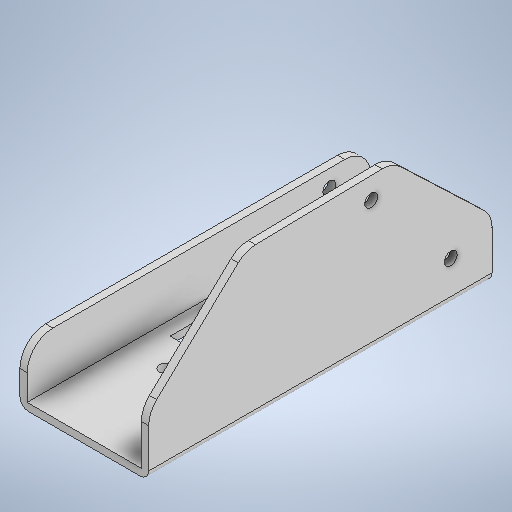
# Autodesk Inventor part: gripper servo mount
Saved by Autodesk Inventor 2025.2 (Build 292293000, 293)
## iProperties
Created: 2025-05-22
Part Number: gripper servo mount
Material: Generic
Document SubType Name: Modeling
Designer: Verchasv
Density: 1 g/cm^3
Appearance: Default
Author: Verchasv
Autodesk Inventor part; units mm, degrees
ref_plane "YZ Plane" through (0, 0, 0) normal (1, 0, 0) x (0, 1, 0)
ref_plane "XZ Plane" through (0, 0, 0) normal (0, 1, 0) x (-1, 0, 0)
ref_plane "XY Plane" through (0, 0, 0) normal (0, 0, 1) x (1, 0, 0)
sketch "Sketch1" plane through (0, 0, 0) normal (0, 1, 0) x (-1, 0, 0)
  line L0 (0, 0) -> (20, 0)
  line L1 (20, 0) -> (20, -40)
  line L2 (20, -40) -> (0, -40)
  line L3 (0, -40) -> (0, 0)
  line L4 (25, 30) -> (-5, 30)
  line L5 (-5, 30) -> (-5, -50)
  line L6 (-5, -50) -> (25, -50)
  line L7 (25, -50) -> (25, 30)
  dimension "d0" = 20
  dimension "d1" = 40
  dimension "d2" = 30
  dimension "d3" = 30
  dimension "d4" = 10
  dimension "d5" = 5
  constraints: 16 end point, 4 parallel, 2 horizontal, 2 perpendicular
  measures "d0" distance of L1.end L2.end
  measures "d1" distance of L0.end L1.end
  measures "d2" distance of L4.start L4.end
  measures "d3" distance between parallel lines of L0 L4
  measures "d4" distance between parallel lines of L2 L6
  measures "d5" distance between parallel lines of L5 L3
extrude "Extrusion1" add sketch "Sketch1" along normal blind 1.7
sketch "Sketch2" plane through (5, 0, 30) normal (1, 0, 0) x (0, 0, -1)
  line L0 (0, 0) -> (0, 1.7) projected
  line L1 (0, 1.7) -> (0, 13.7)
  line L2 (0, 13.7) -> (22.5503, 35.1708)
  line L3 (22.5503, 35.1708) -> (56.8462, 35.7913)
  line L4 (56.8462, 35.7913) -> (80, 13.7)
  line L5 (80, 0) -> (80, 1.7) projected
  line L6 (80, 13.7) -> (80, 1.7)
  line L7 (0, 1.7) -> (80, 1.7) projected
  circle A0 centre (70.3665, 9.7) radius 1.5
  circle A1 centre (70.3665, 9.7) radius 28
  line L8 (24.8863, 30.7) -> (59.3173, 30.7)
  circle A2 centre (51.8462, 30.7) radius 1.5
  point P0 (30, 0)
  dimension "d11" = 56
  dimension "d8" = 0
  dimension "d9" = 3
  dimension "d10" = 8
  dimension "d12" = 29
  dimension "d13" = 3
  dimension "d14" = 5
  dimension "d15" = 5
  dimension "d16" = 12
  dimension "d19" = 12
  constraints: 12 end point, 2 centre point, 1 coincident, 1 horizontal, 1 point on line, 1 vertical, 3 other
  measures "d8" horizontal distance of L5.end L4.end
  measures "d9" diameter of A0
  measures "d10" distance from line of L7 A0.centre
  measures "d12" distance between parallel lines of L7 L8
  measures "d13" diameter of A2
  measures "d14" horizontal distance of L3.end A2.centre
  measures "d15" distance from line of L3 A2.centre
  measures "d16" distance of L4.end L5.end
  measures "d19" distance of L0.end L1.end
extrude "Extrusion2" add sketch "Sketch2" against normal blind 1.7 contours L1 L2 L3 L4 A1 A2 L7 | A1 A2 L4 L6 L7
sketch "Sketch3" plane through (-25, 0, -50) normal (-1, 0, 0) x (0, 0, 1)
  line L0 (0, 0) -> (0, 13.7) projected
  line L1 (23.1538, 35.7913) -> (0, 13.7) projected
  line L2 (0, 1.667) -> (0, 13.7)
  line L3 (0, 13.7) -> (80, 13.7)
  line L4 (80, 1.7) -> (0, 1.7) projected
  line L5 (80, 0) -> (80, 1.7) projected
  line L6 (0, 1.7) -> (80, 1.7)
  line L7 (80, 1.7) -> (80, 13.7)
  circle A0 centre (9.6335, 9.7) radius 1.5 projected
  circle A1 centre (9.6335, 9.7) radius 1.5
  point P0 (50, 0)
  dimension "d20" = 80
  dimension "d21" = 3
  constraints: 8 end point, 1 centre point, 1 coincident, 1 horizontal, 1 perpendicular, 1 point on line, 1 vertical
  measures "d20" distance of L0.end L3.end
  measures "d21" diameter of A1
extrude "Extrusion3" add sketch "Sketch3" against normal blind 1.7
fillet "Fillet1" radius 2 2 edges at (-25, 0, -10) (5, 0, -10)
fillet "Fillet2" radius 6 6 edges at (4.15, 13.7, 30) (4.15, 35.1708, 7.4497) (4.15, 35.7913, -26.8462) (4.15, 13.7, -50) (-24.15, 13.7, -50) (-24.15, 13.7, 30)
sketch "Sketch4" plane through (0, 1.7, 0) normal (0, 1, 0) x (1, 0, 0)
  line L0 (-6, 47) -> (-14, 47)
  line L1 (-14, 47) -> (-14, -7)
  line L2 (-14, -7) -> (-6, -7)
  line L3 (-6, -7) -> (-6, 47)
  line L4 (-20, 0) -> (-20, 40) projected
  line L5 (-20, 40) -> (0, 40) projected
  circle A0 centre (-6, 47) radius 1.5
  circle A1 centre (-14, 47) radius 1.5
  circle A2 centre (-6, -7) radius 1.5
  circle A3 centre (-14, -7) radius 1.5
  point P0 (0, 0)
  point P1 (-10, 40)
  dimension "d26" = 8
  dimension "d27" = 54
  dimension "d28" = 6
  dimension "d29" = 7
  dimension "d30" = 3
  dimension "d31" = 3
  dimension "d32" = 3
  dimension "d33" = 3
  constraints: 8 end point, 4 centre point, 4 coincident, 2 parallel, 1 horizontal, 1 midpoint, 1 perpendicular
  measures "d26" distance of L2.end L1.end
  measures "d27" distance of L1.end L0.end
  measures "d28" distance between parallel lines of L4 L1
  measures "d29" distance from line of point (-10, 40) L0
  measures "d30" diameter of A0
  measures "d31" diameter of A1
  measures "d32" diameter of A2
  measures "d33" diameter of A3
extrude "Extrusion4" cut sketch "Sketch4" against normal through all contours A1 L1 L0 | L0 L1 A1 | A0 L3 L0 | L0 L3 A0 | A3 L2 L1 | L1 L2 A3 | A2 L2 L3 | L3 L2 A2
body "Solid1"
